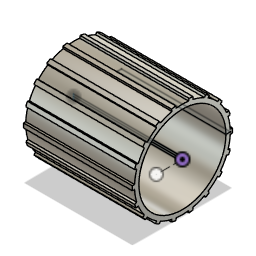
straight bars + spokes v6 (Autodesk Fusion 360 archive; units mm, degrees)
design "straight bar tread"
Autodesk Fusion 360 part; units mm, degrees
note: some values were not read from the file. Chosen so that the rebuilt part matches the saved one: which bodies a step acts on.
sketch "Sketch1" plane through (0, 0, 0) normal (0, 1, 0) x (1, 0, 0) in component "tread"
  line L0 (-50, 22) -> (0, 22)
  line L1 (0, 22) -> (0, 20)
  line L2 (0, 20) -> (-50, 20)
  line L3 (-50, 20) -> (-50, 22)
  line L4 (0, 0) -> (0, -12) construction
  dimension "d1" = 50
  dimension "d2" = 2
  dimension "d3" = 20
  constraint horizontal L0
  constraint vertical L1
  constraint horizontal L2
  constraint vertical L3
  constraint coincident L4.start origin
  constraint vertical L4
  constraint collinear L1 L4
  measures "d1" distance of L1.end L2.end
  measures "d2" distance of L0.end L1.end
  measures "d3" distance of L4.start L1.end
revolve "Revolve1" add sketch "Sketch1" angle 360 about axis through (1.75, 0, 0) along (1, 0, 0) makes body 1 in component "tread"
sketch "Sketch2" plane through (0, 0, 0) normal (0, 0, 1) x (1, 0, 0) in component "tread"
  line L0 (0, 0) -> (-50, 0)
  line L1 (0, 1) -> (-50, 1)
  line L2 (0, -1) -> (-50, -1)
  line L3 (0, -1) -> (0, 1)
  line L4 (-50, -1) -> (-50, 1)
  dimension "d5" = 50
  dimension "d6" = 1
  dimension "d7" = -1
  constraint coincident L0.start origin
  constraint horizontal L0
  constraint perpendicular L1 L3
  constraint perpendicular L1 L4
  measures "d5" distance of L0.start L0.end
extrude "Extrude1" add sketch "Sketch2" along normal mid plane 46 separate body makes body 2 in component "tread"
pattern_circular "C-Pattern1" count 9 over 360 about axis through (1.75, 0, 0) along (1, 0, 0) of "Extrude1" makes body 3 makes body 4 makes body 5 makes body 6 makes body 7 makes body 8 makes body 9 makes body 10 in component "tread"
sketch "Sketch3" plane through (0, 0, 0) normal (1, 0, 0) x (0, 0, -1) in component "tread"
  circle A0 centre (0, 0) radius 20
  dimension "d14" = 40
  constraint coincident A0.centre origin
  measures "d14" diameter of A0
extrude "Extrude2" cut sketch "Sketch3" against normal blind 50 bodies 2 makes body 11 at (-16.6667, 1, -20.9833) in component "tread"
extrude "Extrude3" cut sketch "Sketch3" against normal blind 50 bodies 3 4 5 6 7 8 9 10 makes body 19 at (-16.6667, -13.3699, -17.4894) makes body 18 at (-33.3333, -20.4909, -4.6285) makes body 17 at (-33.3333, -18.6721, 9.6256) makes body 16 at (-16.6667, -8.4613, 20.3234) makes body 15 at (-33.3333, -8.4613, -20.3234) makes body 14 at (-33.3333, -18.6721, -9.6256) makes body 13 at (-33.3333, -21.4839, 4.8036) makes body 12 at (-16.6667, -12.7218, 16.7169) in component "tread"
combine "Combine1" operation add target body 1 tool bodies 5 in component "tread"
combine "Combine2" operation add target body 1 tool bodies 3 4 8 6 7 9 10 13 12 11 18 19 2 16 15 14 17 in component "tread"
component "tread" placed x (1, 0, 0) y (0, 1, 0) z (0, 0, 1) at (0, 0, 0)
